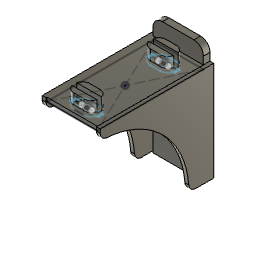
rack_mount_foot (Autodesk Fusion 360 design; units mm, degrees)
Autodesk Fusion 360 part; units mm, degrees
sketch "Sketch1" plane through (0, 0, 0) normal (0, 0, 1) x (1, 0, 0)
  line L0 (10.65, 22.4) -> (-10.65, 22.4)
  line L1 (-10.65, 22.4) -> (-10.65, -22.4)
  line L2 (-10.65, -22.4) -> (10.65, -22.4)
  line L3 (10.65, -22.4) -> (10.65, 22.4)
  line L4 (10.65, 22.4) -> (-10.65, -22.4) construction
  line L5 (-10.65, 22.4) -> (10.65, -22.4) construction
  line L6 (2.11, -19.55) -> (-2.11, -19.55)
  line L7 (-5.4, -16.26) -> (-5.4, -16.15)
  line L8 (-2, -12.75) -> (2, -12.75)
  line L9 (5.4, -16.15) -> (5.4, -16.26)
  line L10 (5.4, -19.55) -> (-5.4, -12.75) construction
  line L11 (-5.4, -19.55) -> (5.4, -12.75) construction
  line L12 (2.1277, 12.7404) -> (-2.0179, 12.7404)
  line L13 (-5.4179, 16.1382) -> (-5.4179, 16.138)
  line L14 (-2.0179, 19.5402) -> (2.0175, 19.5402)
  line L15 (5.4175, 16.1453) -> (5.4176, 16.0353)
  line L16 (5.4226, 12.7404) -> (-5.3876, 19.5402) construction
  line L17 (-5.439, 12.7404) -> (5.4124, 19.5402) construction
  arc A0 (-2.0179, 19.5402) -> (-5.4179, 16.138) centre (-2.0179, 16.1402) ccw
  arc A1 (-5.4179, 16.1382) -> (-2.0179, 12.7404) centre (-2.0179, 16.1404) ccw
  arc A2 (5.4175, 16.1453) -> (2.0175, 19.5402) centre (2.0175, 16.1402) ccw
  arc A3 (2.1277, 12.7404) -> (5.4176, 16.0353) centre (2.1277, 16.0304) ccw
  arc A4 (-2, -12.75) -> (-5.4, -16.15) centre (-2, -16.15) ccw
  arc A5 (5.4, -16.15) -> (2, -12.75) centre (2, -16.15) ccw
  arc A6 (-5.4, -16.26) -> (-2.11, -19.55) centre (-2.11, -16.26) ccw
  arc A7 (2.11, -19.55) -> (5.4, -16.26) centre (2.11, -16.26) ccw
  line L18 (6, 15.2) -> (-6, 15.2)
  line L19 (-6, 15.2) -> (-6, 17.2)
  line L20 (-6, 17.2) -> (6, 17.2)
  line L21 (6, 17.2) -> (6, 15.2)
  line L22 (6, 15.2) -> (-6, 17.2) construction
  line L23 (-6, 15.2) -> (6, 17.2) construction
  line L24 (6, -17.2) -> (-6, -17.2)
  line L25 (-6, -17.2) -> (-6, -15.2)
  line L26 (-6, -15.2) -> (6, -15.2)
  line L27 (6, -15.2) -> (6, -17.2)
  line L28 (6, -17.2) -> (-6, -15.2) construction
  line L29 (-6, -17.2) -> (6, -15.2) construction
  point P0 (0, -16.15)
  point P1 (0.0021, 16.15)
  point P2 (0, 16.2)
  point P3 (0, -16.2)
  dimension "d1" = 21.3
  dimension "d2" = 44.8
  dimension "d3" = 10.8
  dimension "d4" = 6.8
  dimension "d5" = 6.25
  dimension "d6" = 10.8
  dimension "d7" = 6.8
  dimension "d8" = 6.25
  dimension "d9" = 3.4
  dimension "d10" = 3.4
  dimension "d11" = 3.4
  dimension "d12" = 3.29
  dimension "d13" = 3.4
  dimension "d14" = 3.4
  dimension "d15" = 3.29
  dimension "d16" = 3.29
  dimension "d17" = 2
  dimension "d18" = 2
  constraint horizontal L0
  constraint perpendicular L0 L1
  constraint parallel L0 L2
  constraint parallel L1 L3
  constraint coincident L4 origin
  constraint coincident L5 origin
  constraint horizontal L6
  constraint perpendicular L6 L7
  constraint parallel L6 L8
  constraint parallel L7 L9
  constraint coincident L10 P0
  constraint coincident L11 P0
  constraint horizontal L12
  constraint parallel L12 L14
  constraint coincident L16 P1
  constraint coincident L17 P1
  constraint coincident L16.end L14
  constraint tangent L14 A0
  constraint coincident L17.start L13
  constraint coincident L17.start L12
  constraint tangent L12 A1
  constraint coincident L17.end L14
  constraint coincident L17.end L15
  constraint tangent L14 A2
  constraint tangent L15 A2
  constraint coincident L16.start L15
  constraint coincident L16.start L12
  constraint tangent L15 A3
  constraint tangent L12 A3
  constraint coincident L10.end L7
  constraint coincident L10.end L8
  constraint tangent L7 A4
  constraint tangent L8 A4
  constraint coincident L11.end L8
  constraint coincident L11.end L9
  constraint tangent L8 A5
  constraint tangent L9 A5
  constraint coincident L11.start L7
  constraint coincident L11.start L6
  constraint tangent L7 A6
  constraint tangent L6 A6
  constraint coincident L10.start L6
  constraint coincident L10.start L9
  constraint tangent L6 A7
  constraint tangent L9 A7
  constraint horizontal L18
  constraint perpendicular L18 L19
  constraint parallel L18 L20
  constraint parallel L19 L21
  constraint coincident L22 P2
  constraint coincident L23 P2
  constraint horizontal L24
  constraint perpendicular L24 L25
  constraint parallel L24 L26
  constraint parallel L25 L27
  constraint coincident L28 P3
  constraint coincident L29 P3
  measures "d1" distance of L1.end L2.end
  measures "d2" distance of L0.end L1.end
  measures "d3" distance of L10.end L11.end
  measures "d4" distance of L11.start L10.end
  measures "d5" distance of L2 P0
  measures "d6" distance of L16.end L17.end
  measures "d7" distance of L17.start L16.end
  measures "d8" distance of L0 P1
  measures "d9" radius of A0
  measures "d10" radius of A1
  measures "d11" radius of A2
  measures "d12" radius of A3
  measures "d13" radius of A4
  measures "d14" radius of A5
  measures "d15" radius of A6
  measures "d16" radius of A7
  measures "d17" distance of L18.end L19.end
  measures "d18" distance of L24.end L25.end
extrude "Extrude2" add sketch "Sketch1" along normal blind 6 contours L6 A6 A7 L24 | L8 A4 A5 L26 | L12 A1 A3 L18 | L14 A0 A2 L20 makes body 1 at (-1.7496, 17.2, 2) makes body 2 at (-1.7549, -15.2, 2) makes body 3 at (1.779, 15.2, 2) makes body 4 at (-1.7543, -17.2, 4)
extrude "Extrude1" add sketch "Sketch1" along normal blind 1.6 separate body makes body 5
sketch "Sketch2" plane through (0, -19.55, 0) normal (0, -1, 0) x (1, 0, 0)
  line L0 (-2.11, 0) -> (2.11, 0)
  line L1 (2.11, 0) -> (2.11, 6)
  line L2 (2.11, 6) -> (-2.11, 6)
  line L3 (-2.11, 6) -> (-2.11, 0)
  line L4 (1.2, 2.8) -> (-1.2, 2.8)
  line L5 (-1.2, 2.8) -> (-1.2, 5.2)
  line L6 (-1.2, 5.2) -> (1.2, 5.2)
  line L7 (1.2, 5.2) -> (1.2, 2.8)
  line L8 (1.2, 2.8) -> (-1.2, 5.2) construction
  line L9 (-1.2, 2.8) -> (1.2, 5.2) construction
  point P0 (0, 4)
  dimension "d23" = 2.4
  dimension "d24" = 2.4
  constraint horizontal L4
  constraint perpendicular L4 L5
  constraint parallel L4 L6
  constraint parallel L5 L7
  constraint coincident L8 P0
  constraint coincident L9 P0
  measures "d23" distance of L5.end L6.end
  measures "d24" distance of L4.end L5.end
extrude "Extrude3" add sketch "Sketch2" along normal blind 0.8 draft -45 contours L4 L5 L6 L7 bodies 4
sketch "Sketch3" plane through (0, 19.5402, 0) normal (0, 1, 0) x (-1, 0, 0)
  line L0 (-2.0175, 0) -> (2.0179, 0)
  line L1 (2.0179, 0) -> (2.0179, 6)
  line L2 (2.0179, 6) -> (-2.0175, 6)
  line L3 (-2.0175, 6) -> (-2.0175, 0)
  line L4 (1.2, 2.8) -> (-1.2, 2.8)
  line L5 (-1.2, 2.8) -> (-1.2, 5.2)
  line L6 (-1.2, 5.2) -> (1.2, 5.2)
  line L7 (1.2, 5.2) -> (1.2, 2.8)
  line L8 (1.2, 2.8) -> (-1.2, 5.2) construction
  line L9 (-1.2, 2.8) -> (1.2, 5.2) construction
  point P0 (0, 4)
  dimension "d27" = 2.4
  dimension "d28" = 2.4
  constraint horizontal L4
  constraint perpendicular L4 L5
  constraint parallel L4 L6
  constraint parallel L5 L7
  constraint coincident L8 P0
  constraint coincident L9 P0
  measures "d27" distance of L5.end L6.end
  measures "d28" distance of L4.end L5.end
extrude "Extrude4" add sketch "Sketch3" along normal blind 0.8 draft -45 contours L4 L5 L6 L7 bodies 1
sketch "Sketch4" plane through (0, 22.4, 0) normal (0, 1, 0) x (-1, 0, 0)
  line L0 (-10.65, 0) -> (10.65, 0)
  line L1 (10.65, 0) -> (10.65, 1.6)
  line L2 (10.65, 1.6) -> (-10.65, 1.6)
  line L3 (-10.65, 1.6) -> (-10.65, 0)
  line L4 (-10.65, 8.8406) -> (10.65, 8.8406)
  line L5 (10.65, 8.8406) -> (10.65, -41.1594)
  line L6 (10.65, -41.1594) -> (-10.65, -41.1594)
  line L7 (-10.65, -41.1594) -> (-10.65, 8.8406)
  dimension "d31" = 21.3
  dimension "d32" = 50
  constraint horizontal L4
  constraint vertical L5
  constraint horizontal L6
  constraint vertical L7
  measures "d31" distance of L4.start L4.end
  measures "d32" distance of L4.start L6.end
extrude "Extrude5" add sketch "Sketch4" along normal blind 2.8 bodies 5
sketch "Sketch5" plane through (-10.65, 0, 0) normal (-1, 0, 0) x (0, -1, 0)
  line L0 (-22.4, 0) -> (22.4, 0)
  line L1 (22.4, 0) -> (22.4, 1.6)
  line L2 (22.4, 1.6) -> (-22.4, 1.6)
  line L3 (-22.4, 1.6) -> (-22.4, 8.8406)
  line L4 (-22.4, 8.8406) -> (-25.2, 8.8406)
  line L5 (-25.2, 8.8406) -> (-25.2, -41.1594)
  line L6 (-25.2, -41.1594) -> (-22.4, -41.1594)
  line L7 (-22.4, -41.1594) -> (-22.4, 0)
  line L8 (-25.2, 1.6) -> (22.8, 1.6)
  line L9 (22.8, 1.6) -> (22.8, -40.4)
  line L10 (22.8, -40.4) -> (-25.2, -40.4)
  line L11 (-25.2, -40.4) -> (-25.2, 1.6)
  circle A0 centre (22.8, -40.4) radius 37.5
  dimension "d35" = 48
  dimension "d36" = 42
  dimension "d37" = 75
  constraint horizontal L8
  constraint vertical L9
  constraint horizontal L10
  constraint vertical L11
  constraint coincident L5 L8.start
  constraint coincident L9.end L10.start
  measures "d35" distance of L8.start L8.end
  measures "d36" distance of L8.start L10.end
  measures "d37" diameter of A0
extrude "Extrude6" add sketch "Sketch5" along normal blind 1.6 contours L0 L1 L2 L5 L7 L8 L10 L11 | L0 L1 L7 L8 L9 L10 A0 bodies 5
sketch "Sketch6" plane through (10.65, 0, 0) normal (1, 0, 0) x (0, 1, 0)
  line L0 (-22.4, 0) -> (22.4, 0)
  line L1 (22.4, 0) -> (22.4, -41.1594)
  line L2 (22.4, -41.1594) -> (25.2, -41.1594)
  line L3 (25.2, -41.1594) -> (25.2, 8.8406)
  line L4 (25.2, 8.8406) -> (22.4, 8.8406)
  line L5 (22.4, 8.8406) -> (22.4, 1.6)
  line L6 (22.4, 1.6) -> (-22.4, 1.6)
  line L7 (-22.4, 1.6) -> (-22.4, 0)
  line L8 (25.2, 1.6369) -> (-22.8, 1.6369)
  line L9 (-22.8, 1.6369) -> (-22.8, -40.3631)
  line L10 (-22.8, -40.3631) -> (25.2, -40.3631)
  line L11 (25.2, -40.3631) -> (25.2, 1.6369)
  circle A0 centre (-22.8, -40.3631) radius 37.5
  dimension "d40" = 48
  dimension "d41" = 42
  dimension "d42" = 75
  constraint horizontal L8
  constraint vertical L9
  constraint horizontal L10
  constraint vertical L11
  constraint coincident L3 L8.start
  constraint coincident L9.end L10.start
  measures "d40" distance of L8.start L8.end
  measures "d41" distance of L8.start L10.end
  measures "d42" diameter of A0
extrude "Extrude7" add sketch "Sketch6" along normal blind 1.6 contours L0 L1 L3 L5 L6 L7 L8 L10 L11 | L0 L1 L5 L6 L7 L8 L9 L10 A0 bodies 5
fillet "Fillet1" radius 3 2 edges at (-11.45, 14.7, -40.4) (-11.45, -22.8, -2.9) on bodies 5
fillet "Fillet2" radius 3 2 edges at (11.45, 14.7, -40.3631) (11.45, -22.8, -2.8631) on bodies 5
fillet "Fillet3" radius 4 2 edges at (10.65, 23.8, 8.8406) (-10.65, 23.8, 8.8406) on bodies 5
